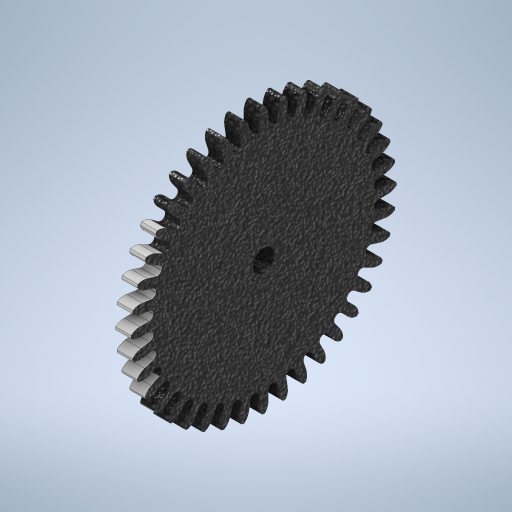
# Autodesk Inventor part: Rear_tubo
Saved by Autodesk Inventor 2024 (Build 280153020, 153B)
## iProperties
Created: 2023-05-22
Part Number: Rear_tubo
Material: Generic
Document SubType Name: Modeling
Designer: Diego
Density: 1 g/cm^3
Appearance: Default
Author: Diego
Autodesk Inventor part; units mm, degrees
ref_plane "YZ Plane" through (0, 0, 0) normal (1, 0, 0) x (0, 1, 0)
ref_plane "XZ Plane" through (0, 0, 0) normal (0, 1, 0) x (-1, 0, 0)
ref_plane "XY Plane" through (0, 0, 0) normal (0, 0, 1) x (1, 0, 0)
sketch "Sketch1" plane through (0, 0, 0) normal (1, 0, 0) x (0, 1, 0)
  circle A0 centre (0, 0) radius 2.5
  arc A1 (-27.9137, 2.1969) -> (-27.9137, -2.1969) centre (0, 0) ccw construction
  line L0 (0, 0) -> (38.0668, 0) construction
  line L1 (0, 0) -> (36.3288, -2.8591) construction
  line L2 (0, 0) -> (35.2598, 2.775) construction
  line L3 (25.9214, 1.02) -> (27.9814, 1.02)
  line L4 (25.9214, -1.02) -> (27.9814, -1.02)
  arc A2 (29.9985, 0.3) -> (27.9814, 1.02) centre (28.0479, -1.9793) ccw
  arc A3 (27.9814, -1.02) -> (29.9985, -0.3) centre (28.0479, 1.9793) ccw
  arc A4 (29.9985, -0.3) -> (29.9985, 0.3) centre (0, 0) ccw
  arc A5 (-29.9985, 0.3) -> (-29.9985, -0.3) centre (0, 0) ccw
  arc A6 (25.9214, -1.02) -> (24.9244, -1.9423) centre (25.9214, -2.02) ccw
  arc A7 (24.9244, 1.9423) -> (25.9214, 1.02) centre (25.9214, 2.02) ccw
  arc A8 (24.3137, 5.8174) -> (25.4427, 5.0624) centre (25.2863, 6.0501) ccw
  line L5 (25.4427, 5.0624) -> (27.4774, 5.3847)
  arc A9 (25.7618, 3.0476) -> (24.9214, 1.9806) centre (25.9183, 2.0599) ccw
  arc A10 (27.7965, 3.3698) -> (29.6761, 4.3965) centre (27.3929, 6.3425) ccw
  arc A11 (29.6761, 4.3965) -> (29.5822, 4.9891) centre (0, 0) ccw
  arc A12 (29.5822, 4.9891) -> (27.4774, 5.3847) centre (28.0122, 2.4328) ccw
  line L6 (25.7618, 3.0476) -> (27.7965, 3.3698)
  arc A13 (23.1043, 9.5493) -> (24.3375, 8.9802) centre (24.0285, 9.9313) ccw
  line L7 (24.3375, 8.9802) -> (26.2967, 9.6168)
  arc A14 (24.9679, 7.0401) -> (24.3048, 5.8548) centre (25.2769, 6.089) ccw
  arc A15 (26.9271, 7.6767) -> (28.623, 8.9847) centre (26.0635, 10.5497) ccw
  arc A16 (28.623, 8.9847) -> (28.4376, 9.5554) centre (0, 0) ccw
  arc A17 (28.4376, 9.5554) -> (26.2967, 9.6168) centre (27.2867, 6.7849) ccw
  line L8 (24.9679, 7.0401) -> (26.9271, 7.6767)
  arc A18 (21.326, 13.0461) -> (22.6331, 12.6769) centre (22.1791, 13.5679) ccw
  line L9 (22.6331, 12.6769) -> (24.4686, 13.6121)
  arc A19 (23.5592, 10.8592) -> (23.0896, 9.5848) centre (24.0132, 9.9682) ccw
  arc A20 (25.3947, 11.7945) -> (26.8651, 13.3517) centre (24.0923, 14.497) ccw
  arc A21 (26.8651, 13.3517) -> (26.5927, 13.8863) centre (0, 0) ccw
  arc A22 (26.5927, 13.8863) -> (24.4686, 13.6121) centre (25.8894, 10.9699) ccw
  line L10 (23.5592, 10.8592) -> (25.3947, 11.7945)
  arc A23 (19.0226, 16.2216) -> (20.3713, 16.0614) centre (19.7835, 16.8704) ccw
  line L11 (20.3713, 16.0614) -> (22.0379, 17.2723)
  arc A24 (21.5704, 14.411) -> (21.306, 13.0789) centre (22.1582, 13.602) ccw
  arc A25 (23.237, 15.6219) -> (24.4456, 17.39) centre (21.5278, 18.0874) ccw
  arc A26 (24.4456, 17.39) -> (24.093, 17.8754) centre (0, 0) ccw
  arc A27 (24.093, 17.8754) -> (22.0379, 17.2723) centre (23.8546, 14.8849) ccw
  line L12 (21.5704, 14.411) -> (23.237, 15.6219)
  arc A28 (16.2508, 18.9977) -> (17.608, 19.0505) centre (16.9009, 19.7576) ccw
  line L13 (17.608, 19.0505) -> (19.0646, 20.5071)
  arc A29 (19.0505, 17.608) -> (18.9977, 16.2508) centre (19.7576, 16.9009) ccw
  arc A30 (20.5071, 19.0646) -> (21.4243, 21) centre (18.4333, 21.2324) ccw
  arc A31 (21.4243, 21) -> (21, 21.4243) centre (0, 0) ccw
  arc A32 (21, 21.4243) -> (19.0646, 20.5071) centre (21.2324, 18.4333) ccw
  line L14 (19.0505, 17.608) -> (20.5071, 19.0646)
  arc A33 (13.0789, 21.306) -> (14.411, 21.5704) centre (13.602, 22.1582) ccw
  line L15 (14.411, 21.5704) -> (15.6219, 23.237)
  arc A34 (16.0614, 20.3713) -> (16.2216, 19.0226) centre (16.8704, 19.7835) ccw
  arc A35 (17.2723, 22.0379) -> (17.8754, 24.093) centre (14.8849, 23.8546) ccw
  arc A36 (17.8754, 24.093) -> (17.39, 24.4456) centre (0, 0) ccw
  arc A37 (17.39, 24.4456) -> (15.6219, 23.237) centre (18.0874, 21.5278) ccw
  line L16 (16.0614, 20.3713) -> (17.2723, 22.0379)
  arc A38 (9.5848, 23.0896) -> (10.8592, 23.5592) centre (9.9682, 24.0132) ccw
  line L17 (10.8592, 23.5592) -> (11.7945, 25.3947)
  arc A39 (12.6769, 22.6331) -> (13.0461, 21.326) centre (13.5679, 22.1791) ccw
  arc A40 (13.6121, 24.4686) -> (13.8863, 26.5927) centre (10.9699, 25.8894) ccw
  arc A41 (13.8863, 26.5927) -> (13.3517, 26.8651) centre (0, 0) ccw
  arc A42 (13.3517, 26.8651) -> (11.7945, 25.3947) centre (14.497, 24.0923) ccw
  line L18 (12.6769, 22.6331) -> (13.6121, 24.4686)
  arc A43 (5.8548, 24.3048) -> (7.0401, 24.9679) centre (6.089, 25.2769) ccw
  line L19 (7.0401, 24.9679) -> (7.6767, 26.9271)
  arc A44 (8.9802, 24.3375) -> (9.5493, 23.1043) centre (9.9313, 24.0285) ccw
  arc A45 (9.6168, 26.2967) -> (9.5554, 28.4376) centre (6.7849, 27.2867) ccw
  arc A46 (9.5554, 28.4376) -> (8.9847, 28.623) centre (0, 0) ccw
  arc A47 (8.9847, 28.623) -> (7.6767, 26.9271) centre (10.5497, 26.0635) ccw
  line L20 (8.9802, 24.3375) -> (9.6168, 26.2967)
  arc A48 (1.9806, 24.9214) -> (3.0476, 25.7618) centre (2.0599, 25.9183) ccw
  line L21 (3.0476, 25.7618) -> (3.3698, 27.7965)
  arc A49 (5.0624, 25.4427) -> (5.8174, 24.3137) centre (6.0501, 25.2863) ccw
  arc A50 (5.3847, 27.4774) -> (4.9891, 29.5822) centre (2.4328, 28.0122) ccw
  arc A51 (4.9891, 29.5822) -> (4.3965, 29.6761) centre (0, 0) ccw
  arc A52 (4.3965, 29.6761) -> (3.3698, 27.7965) centre (6.3425, 27.3929) ccw
  line L22 (5.0624, 25.4427) -> (5.3847, 27.4774)
  arc A53 (-1.9423, 24.9244) -> (-1.02, 25.9214) centre (-2.02, 25.9214) ccw
  line L23 (-1.02, 25.9214) -> (-1.02, 27.9814)
  arc A54 (1.02, 25.9214) -> (1.9423, 24.9244) centre (2.02, 25.9214) ccw
  arc A55 (1.02, 27.9814) -> (0.3, 29.9985) centre (-1.9793, 28.0479) ccw
  arc A56 (0.3, 29.9985) -> (-0.3, 29.9985) centre (0, 0) ccw
  arc A57 (-0.3, 29.9985) -> (-1.02, 27.9814) centre (1.9793, 28.0479) ccw
  line L24 (1.02, 25.9214) -> (1.02, 27.9814)
  arc A58 (-5.8174, 24.3137) -> (-5.0624, 25.4427) centre (-6.0501, 25.2863) ccw
  line L25 (-5.0624, 25.4427) -> (-5.3847, 27.4774)
  arc A59 (-3.0476, 25.7618) -> (-1.9806, 24.9214) centre (-2.0599, 25.9183) ccw
  arc A60 (-3.3698, 27.7965) -> (-4.3965, 29.6761) centre (-6.3425, 27.3929) ccw
  arc A61 (-4.3965, 29.6761) -> (-4.9891, 29.5822) centre (0, 0) ccw
  arc A62 (-4.9891, 29.5822) -> (-5.3847, 27.4774) centre (-2.4328, 28.0122) ccw
  line L26 (-3.0476, 25.7618) -> (-3.3698, 27.7965)
  arc A63 (-9.5493, 23.1043) -> (-8.9802, 24.3375) centre (-9.9313, 24.0285) ccw
  line L27 (-8.9802, 24.3375) -> (-9.6168, 26.2967)
  arc A64 (-7.0401, 24.9679) -> (-5.8548, 24.3048) centre (-6.089, 25.2769) ccw
  arc A65 (-7.6767, 26.9271) -> (-8.9847, 28.623) centre (-10.5497, 26.0635) ccw
  arc A66 (-8.9847, 28.623) -> (-9.5554, 28.4376) centre (0, 0) ccw
  arc A67 (-9.5554, 28.4376) -> (-9.6168, 26.2967) centre (-6.7849, 27.2867) ccw
  line L28 (-7.0401, 24.9679) -> (-7.6767, 26.9271)
  arc A68 (-13.0461, 21.326) -> (-12.6769, 22.6331) centre (-13.5679, 22.1791) ccw
  line L29 (-12.6769, 22.6331) -> (-13.6121, 24.4686)
  arc A69 (-10.8592, 23.5592) -> (-9.5848, 23.0896) centre (-9.9682, 24.0132) ccw
  arc A70 (-11.7945, 25.3947) -> (-13.3517, 26.8651) centre (-14.497, 24.0923) ccw
  arc A71 (-13.3517, 26.8651) -> (-13.8863, 26.5927) centre (0, 0) ccw
  arc A72 (-13.8863, 26.5927) -> (-13.6121, 24.4686) centre (-10.9699, 25.8894) ccw
  line L30 (-10.8592, 23.5592) -> (-11.7945, 25.3947)
  arc A73 (-16.2216, 19.0226) -> (-16.0614, 20.3713) centre (-16.8704, 19.7835) ccw
  line L31 (-16.0614, 20.3713) -> (-17.2723, 22.0379)
  arc A74 (-14.411, 21.5704) -> (-13.0789, 21.306) centre (-13.602, 22.1582) ccw
  arc A75 (-15.6219, 23.237) -> (-17.39, 24.4456) centre (-18.0874, 21.5278) ccw
  arc A76 (-17.39, 24.4456) -> (-17.8754, 24.093) centre (0, 0) ccw
  arc A77 (-17.8754, 24.093) -> (-17.2723, 22.0379) centre (-14.8849, 23.8546) ccw
  line L32 (-14.411, 21.5704) -> (-15.6219, 23.237)
  arc A78 (-18.9977, 16.2508) -> (-19.0505, 17.608) centre (-19.7576, 16.9009) ccw
  line L33 (-19.0505, 17.608) -> (-20.5071, 19.0646)
  arc A79 (-17.608, 19.0505) -> (-16.2508, 18.9977) centre (-16.9009, 19.7576) ccw
  arc A80 (-19.0646, 20.5071) -> (-21, 21.4243) centre (-21.2324, 18.4333) ccw
  arc A81 (-21, 21.4243) -> (-21.4243, 21) centre (0, 0) ccw
  arc A82 (-21.4243, 21) -> (-20.5071, 19.0646) centre (-18.4333, 21.2324) ccw
  line L34 (-17.608, 19.0505) -> (-19.0646, 20.5071)
  arc A83 (-21.306, 13.0789) -> (-21.5704, 14.411) centre (-22.1582, 13.602) ccw
  line L35 (-21.5704, 14.411) -> (-23.237, 15.6219)
  arc A84 (-20.3713, 16.0614) -> (-19.0226, 16.2216) centre (-19.7835, 16.8704) ccw
  arc A85 (-22.0379, 17.2723) -> (-24.093, 17.8754) centre (-23.8546, 14.8849) ccw
  arc A86 (-24.093, 17.8754) -> (-24.4456, 17.39) centre (0, 0) ccw
  arc A87 (-24.4456, 17.39) -> (-23.237, 15.6219) centre (-21.5278, 18.0874) ccw
  line L36 (-20.3713, 16.0614) -> (-22.0379, 17.2723)
  arc A88 (-23.0896, 9.5848) -> (-23.5592, 10.8592) centre (-24.0132, 9.9682) ccw
  line L37 (-23.5592, 10.8592) -> (-25.3947, 11.7945)
  arc A89 (-22.6331, 12.6769) -> (-21.326, 13.0461) centre (-22.1791, 13.5679) ccw
  arc A90 (-24.4686, 13.6121) -> (-26.5927, 13.8863) centre (-25.8894, 10.9699) ccw
  arc A91 (-26.5927, 13.8863) -> (-26.8651, 13.3517) centre (0, 0) ccw
  arc A92 (-26.8651, 13.3517) -> (-25.3947, 11.7945) centre (-24.0923, 14.497) ccw
  line L38 (-22.6331, 12.6769) -> (-24.4686, 13.6121)
  arc A93 (-24.3048, 5.8548) -> (-24.9679, 7.0401) centre (-25.2769, 6.089) ccw
  line L39 (-24.9679, 7.0401) -> (-26.9271, 7.6767)
  arc A94 (-24.3375, 8.9802) -> (-23.1043, 9.5493) centre (-24.0285, 9.9313) ccw
  arc A95 (-26.2967, 9.6168) -> (-28.4376, 9.5554) centre (-27.2867, 6.7849) ccw
  arc A96 (-28.4376, 9.5554) -> (-28.623, 8.9847) centre (0, 0) ccw
  arc A97 (-28.623, 8.9847) -> (-26.9271, 7.6767) centre (-26.0635, 10.5497) ccw
  line L40 (-24.3375, 8.9802) -> (-26.2967, 9.6168)
  arc A98 (-24.9214, 1.9806) -> (-25.7618, 3.0476) centre (-25.9183, 2.0599) ccw
  line L41 (-25.7618, 3.0476) -> (-27.7965, 3.3698)
  arc A99 (-25.4427, 5.0624) -> (-24.3137, 5.8174) centre (-25.2863, 6.0501) ccw
  arc A100 (-27.4774, 5.3847) -> (-29.5822, 4.9891) centre (-28.0122, 2.4328) ccw
  arc A101 (-29.5822, 4.9891) -> (-29.6761, 4.3965) centre (0, 0) ccw
  arc A102 (-29.6761, 4.3965) -> (-27.7965, 3.3698) centre (-27.3929, 6.3425) ccw
  line L42 (-25.4427, 5.0624) -> (-27.4774, 5.3847)
  arc A103 (-24.9244, -1.9423) -> (-25.9214, -1.02) centre (-25.9214, -2.02) ccw
  line L43 (-25.9214, -1.02) -> (-27.9814, -1.02)
  arc A104 (-25.9214, 1.02) -> (-24.9244, 1.9423) centre (-25.9214, 2.02) ccw
  arc A105 (-27.9814, 1.02) -> (-29.9985, 0.3) centre (-28.0479, -1.9793) ccw
  arc A106 (-29.9985, 0.3) -> (-29.9985, -0.3) centre (0, 0) ccw
  arc A107 (-29.9985, -0.3) -> (-27.9814, -1.02) centre (-28.0479, 1.9793) ccw
  line L44 (-25.9214, 1.02) -> (-27.9814, 1.02)
  arc A108 (-24.3137, -5.8174) -> (-25.4427, -5.0624) centre (-25.2863, -6.0501) ccw
  line L45 (-25.4427, -5.0624) -> (-27.4774, -5.3847)
  arc A109 (-25.7618, -3.0476) -> (-24.9214, -1.9806) centre (-25.9183, -2.0599) ccw
  arc A110 (-27.7965, -3.3698) -> (-29.6761, -4.3965) centre (-27.3929, -6.3425) ccw
  arc A111 (-29.6761, -4.3965) -> (-29.5822, -4.9891) centre (0, 0) ccw
  arc A112 (-29.5822, -4.9891) -> (-27.4774, -5.3847) centre (-28.0122, -2.4328) ccw
  line L46 (-25.7618, -3.0476) -> (-27.7965, -3.3698)
  arc A113 (-23.1043, -9.5493) -> (-24.3375, -8.9802) centre (-24.0285, -9.9313) ccw
  line L47 (-24.3375, -8.9802) -> (-26.2967, -9.6168)
  arc A114 (-24.9679, -7.0401) -> (-24.3048, -5.8548) centre (-25.2769, -6.089) ccw
  arc A115 (-26.9271, -7.6767) -> (-28.623, -8.9847) centre (-26.0635, -10.5497) ccw
  arc A116 (-28.623, -8.9847) -> (-28.4376, -9.5554) centre (0, 0) ccw
  arc A117 (-28.4376, -9.5554) -> (-26.2967, -9.6168) centre (-27.2867, -6.7849) ccw
  line L48 (-24.9679, -7.0401) -> (-26.9271, -7.6767)
  arc A118 (-21.326, -13.0461) -> (-22.6331, -12.6769) centre (-22.1791, -13.5679) ccw
  line L49 (-22.6331, -12.6769) -> (-24.4686, -13.6121)
  arc A119 (-23.5592, -10.8592) -> (-23.0896, -9.5848) centre (-24.0132, -9.9682) ccw
  arc A120 (-25.3947, -11.7945) -> (-26.8651, -13.3517) centre (-24.0923, -14.497) ccw
  arc A121 (-26.8651, -13.3517) -> (-26.5927, -13.8863) centre (0, 0) ccw
  arc A122 (-26.5927, -13.8863) -> (-24.4686, -13.6121) centre (-25.8894, -10.9699) ccw
  line L50 (-23.5592, -10.8592) -> (-25.3947, -11.7945)
  arc A123 (-19.0226, -16.2216) -> (-20.3713, -16.0614) centre (-19.7835, -16.8704) ccw
  line L51 (-20.3713, -16.0614) -> (-22.0379, -17.2723)
  arc A124 (-21.5704, -14.411) -> (-21.306, -13.0789) centre (-22.1582, -13.602) ccw
  arc A125 (-23.237, -15.6219) -> (-24.4456, -17.39) centre (-21.5278, -18.0874) ccw
  arc A126 (-24.4456, -17.39) -> (-24.093, -17.8754) centre (0, 0) ccw
  arc A127 (-24.093, -17.8754) -> (-22.0379, -17.2723) centre (-23.8546, -14.8849) ccw
  line L52 (-21.5704, -14.411) -> (-23.237, -15.6219)
  arc A128 (-16.2508, -18.9977) -> (-17.608, -19.0505) centre (-16.9009, -19.7576) ccw
  line L53 (-17.608, -19.0505) -> (-19.0646, -20.5071)
  arc A129 (-19.0505, -17.608) -> (-18.9977, -16.2508) centre (-19.7576, -16.9009) ccw
  arc A130 (-20.5071, -19.0646) -> (-21.4243, -21) centre (-18.4333, -21.2324) ccw
  arc A131 (-21.4243, -21) -> (-21, -21.4243) centre (0, 0) ccw
  arc A132 (-21, -21.4243) -> (-19.0646, -20.5071) centre (-21.2324, -18.4333) ccw
  line L54 (-19.0505, -17.608) -> (-20.5071, -19.0646)
  arc A133 (-13.0789, -21.306) -> (-14.411, -21.5704) centre (-13.602, -22.1582) ccw
  line L55 (-14.411, -21.5704) -> (-15.6219, -23.237)
  arc A134 (-16.0614, -20.3713) -> (-16.2216, -19.0226) centre (-16.8704, -19.7835) ccw
  arc A135 (-17.2723, -22.0379) -> (-17.8754, -24.093) centre (-14.8849, -23.8546) ccw
  arc A136 (-17.8754, -24.093) -> (-17.39, -24.4456) centre (0, 0) ccw
  arc A137 (-17.39, -24.4456) -> (-15.6219, -23.237) centre (-18.0874, -21.5278) ccw
  line L56 (-16.0614, -20.3713) -> (-17.2723, -22.0379)
  arc A138 (-9.5848, -23.0896) -> (-10.8592, -23.5592) centre (-9.9682, -24.0132) ccw
  line L57 (-10.8592, -23.5592) -> (-11.7945, -25.3947)
  arc A139 (-12.6769, -22.6331) -> (-13.0461, -21.326) centre (-13.5679, -22.1791) ccw
  arc A140 (-13.6121, -24.4686) -> (-13.8863, -26.5927) centre (-10.9699, -25.8894) ccw
  arc A141 (-13.8863, -26.5927) -> (-13.3517, -26.8651) centre (0, 0) ccw
  arc A142 (-13.3517, -26.8651) -> (-11.7945, -25.3947) centre (-14.497, -24.0923) ccw
  line L58 (-12.6769, -22.6331) -> (-13.6121, -24.4686)
  arc A143 (-5.8548, -24.3048) -> (-7.0401, -24.9679) centre (-6.089, -25.2769) ccw
  line L59 (-7.0401, -24.9679) -> (-7.6767, -26.9271)
  arc A144 (-8.9802, -24.3375) -> (-9.5493, -23.1043) centre (-9.9313, -24.0285) ccw
  arc A145 (-9.6168, -26.2967) -> (-9.5554, -28.4376) centre (-6.7849, -27.2867) ccw
  arc A146 (-9.5554, -28.4376) -> (-8.9847, -28.623) centre (0, 0) ccw
  arc A147 (-8.9847, -28.623) -> (-7.6767, -26.9271) centre (-10.5497, -26.0635) ccw
  line L60 (-8.9802, -24.3375) -> (-9.6168, -26.2967)
  arc A148 (-1.9806, -24.9214) -> (-3.0476, -25.7618) centre (-2.0599, -25.9183) ccw
  line L61 (-3.0476, -25.7618) -> (-3.3698, -27.7965)
  arc A149 (-5.0624, -25.4427) -> (-5.8174, -24.3137) centre (-6.0501, -25.2863) ccw
  arc A150 (-5.3847, -27.4774) -> (-4.9891, -29.5822) centre (-2.4328, -28.0122) ccw
  arc A151 (-4.9891, -29.5822) -> (-4.3965, -29.6761) centre (0, 0) ccw
  arc A152 (-4.3965, -29.6761) -> (-3.3698, -27.7965) centre (-6.3425, -27.3929) ccw
  line L62 (-5.0624, -25.4427) -> (-5.3847, -27.4774)
  arc A153 (1.9423, -24.9244) -> (1.02, -25.9214) centre (2.02, -25.9214) ccw
  line L63 (1.02, -25.9214) -> (1.02, -27.9814)
  arc A154 (-1.02, -25.9214) -> (-1.9423, -24.9244) centre (-2.02, -25.9214) ccw
  arc A155 (-1.02, -27.9814) -> (-0.3, -29.9985) centre (1.9793, -28.0479) ccw
  arc A156 (-0.3, -29.9985) -> (0.3, -29.9985) centre (0, 0) ccw
  arc A157 (0.3, -29.9985) -> (1.02, -27.9814) centre (-1.9793, -28.0479) ccw
  line L64 (-1.02, -25.9214) -> (-1.02, -27.9814)
  arc A158 (5.8174, -24.3137) -> (5.0624, -25.4427) centre (6.0501, -25.2863) ccw
  line L65 (5.0624, -25.4427) -> (5.3847, -27.4774)
  arc A159 (3.0476, -25.7618) -> (1.9806, -24.9214) centre (2.0599, -25.9183) ccw
  arc A160 (3.3698, -27.7965) -> (4.3965, -29.6761) centre (6.3425, -27.3929) ccw
  arc A161 (4.3965, -29.6761) -> (4.9891, -29.5822) centre (0, 0) ccw
  arc A162 (4.9891, -29.5822) -> (5.3847, -27.4774) centre (2.4328, -28.0122) ccw
  line L66 (3.0476, -25.7618) -> (3.3698, -27.7965)
  arc A163 (9.5493, -23.1043) -> (8.9802, -24.3375) centre (9.9313, -24.0285) ccw
  line L67 (8.9802, -24.3375) -> (9.6168, -26.2967)
  arc A164 (7.0401, -24.9679) -> (5.8548, -24.3048) centre (6.089, -25.2769) ccw
  arc A165 (7.6767, -26.9271) -> (8.9847, -28.623) centre (10.5497, -26.0635) ccw
  arc A166 (8.9847, -28.623) -> (9.5554, -28.4376) centre (0, 0) ccw
  arc A167 (9.5554, -28.4376) -> (9.6168, -26.2967) centre (6.7849, -27.2867) ccw
  line L68 (7.0401, -24.9679) -> (7.6767, -26.9271)
  arc A168 (13.0461, -21.326) -> (12.6769, -22.6331) centre (13.5679, -22.1791) ccw
  line L69 (12.6769, -22.6331) -> (13.6121, -24.4686)
  arc A169 (10.8592, -23.5592) -> (9.5848, -23.0896) centre (9.9682, -24.0132) ccw
  arc A170 (11.7945, -25.3947) -> (13.3517, -26.8651) centre (14.497, -24.0923) ccw
  arc A171 (13.3517, -26.8651) -> (13.8863, -26.5927) centre (0, 0) ccw
  arc A172 (13.8863, -26.5927) -> (13.6121, -24.4686) centre (10.9699, -25.8894) ccw
  line L70 (10.8592, -23.5592) -> (11.7945, -25.3947)
  arc A173 (16.2216, -19.0226) -> (16.0614, -20.3713) centre (16.8704, -19.7835) ccw
  line L71 (16.0614, -20.3713) -> (17.2723, -22.0379)
  arc A174 (14.411, -21.5704) -> (13.0789, -21.306) centre (13.602, -22.1582) ccw
  arc A175 (15.6219, -23.237) -> (17.39, -24.4456) centre (18.0874, -21.5278) ccw
  arc A176 (17.39, -24.4456) -> (17.8754, -24.093) centre (0, 0) ccw
  arc A177 (17.8754, -24.093) -> (17.2723, -22.0379) centre (14.8849, -23.8546) ccw
  line L72 (14.411, -21.5704) -> (15.6219, -23.237)
  arc A178 (18.9977, -16.2508) -> (19.0505, -17.608) centre (19.7576, -16.9009) ccw
  line L73 (19.0505, -17.608) -> (20.5071, -19.0646)
  arc A179 (17.608, -19.0505) -> (16.2508, -18.9977) centre (16.9009, -19.7576) ccw
  arc A180 (19.0646, -20.5071) -> (21, -21.4243) centre (21.2324, -18.4333) ccw
  arc A181 (21, -21.4243) -> (21.4243, -21) centre (0, 0) ccw
  arc A182 (21.4243, -21) -> (20.5071, -19.0646) centre (18.4333, -21.2324) ccw
  line L74 (17.608, -19.0505) -> (19.0646, -20.5071)
  arc A183 (21.306, -13.0789) -> (21.5704, -14.411) centre (22.1582, -13.602) ccw
  line L75 (21.5704, -14.411) -> (23.237, -15.6219)
  arc A184 (20.3713, -16.0614) -> (19.0226, -16.2216) centre (19.7835, -16.8704) ccw
  arc A185 (22.0379, -17.2723) -> (24.093, -17.8754) centre (23.8546, -14.8849) ccw
  arc A186 (24.093, -17.8754) -> (24.4456, -17.39) centre (0, 0) ccw
  arc A187 (24.4456, -17.39) -> (23.237, -15.6219) centre (21.5278, -18.0874) ccw
  line L76 (20.3713, -16.0614) -> (22.0379, -17.2723)
  arc A188 (23.0896, -9.5848) -> (23.5592, -10.8592) centre (24.0132, -9.9682) ccw
  line L77 (23.5592, -10.8592) -> (25.3947, -11.7945)
  arc A189 (22.6331, -12.6769) -> (21.326, -13.0461) centre (22.1791, -13.5679) ccw
  arc A190 (24.4686, -13.6121) -> (26.5927, -13.8863) centre (25.8894, -10.9699) ccw
  arc A191 (26.5927, -13.8863) -> (26.8651, -13.3517) centre (0, 0) ccw
  arc A192 (26.8651, -13.3517) -> (25.3947, -11.7945) centre (24.0923, -14.497) ccw
  line L78 (22.6331, -12.6769) -> (24.4686, -13.6121)
  arc A193 (24.3048, -5.8548) -> (24.9679, -7.0401) centre (25.2769, -6.089) ccw
  line L79 (24.9679, -7.0401) -> (26.9271, -7.6767)
  arc A194 (24.3375, -8.9802) -> (23.1043, -9.5493) centre (24.0285, -9.9313) ccw
  arc A195 (26.2967, -9.6168) -> (28.4376, -9.5554) centre (27.2867, -6.7849) ccw
  arc A196 (28.4376, -9.5554) -> (28.623, -8.9847) centre (0, 0) ccw
  arc A197 (28.623, -8.9847) -> (26.9271, -7.6767) centre (26.0635, -10.5497) ccw
  line L80 (24.3375, -8.9802) -> (26.2967, -9.6168)
  arc A198 (24.9214, -1.9806) -> (25.7618, -3.0476) centre (25.9183, -2.0599) ccw
  line L81 (25.7618, -3.0476) -> (27.7965, -3.3698)
  arc A199 (25.4427, -5.0624) -> (24.3137, -5.8174) centre (25.2863, -6.0501) ccw
  arc A200 (27.4774, -5.3847) -> (29.5822, -4.9891) centre (28.0122, -2.4328) ccw
  arc A201 (29.5822, -4.9891) -> (29.6761, -4.3965) centre (0, 0) ccw
  arc A202 (29.6761, -4.3965) -> (27.7965, -3.3698) centre (27.3929, -6.3425) ccw
  line L82 (25.4427, -5.0624) -> (27.4774, -5.3847)
  arc A203 (24.9244, 1.9423) -> (24.9214, 1.9806) centre (0, 0) ccw
  arc A204 (24.3137, 5.8174) -> (24.3048, 5.8548) centre (0, 0) ccw
  arc A205 (23.1043, 9.5493) -> (23.0896, 9.5848) centre (0, 0) ccw
  arc A206 (21.326, 13.0461) -> (21.306, 13.0789) centre (0, 0) ccw
  arc A207 (19.0226, 16.2216) -> (18.9977, 16.2508) centre (0, 0) ccw
  arc A208 (16.2508, 18.9977) -> (16.2216, 19.0226) centre (0, 0) ccw
  arc A209 (13.0789, 21.306) -> (13.0461, 21.326) centre (0, 0) ccw
  arc A210 (9.5848, 23.0896) -> (9.5493, 23.1043) centre (0, 0) ccw
  arc A211 (5.8548, 24.3048) -> (5.8174, 24.3137) centre (0, 0) ccw
  arc A212 (1.9806, 24.9214) -> (1.9423, 24.9244) centre (0, 0) ccw
  arc A213 (-1.9423, 24.9244) -> (-1.9806, 24.9214) centre (0, 0) ccw
  arc A214 (-5.8174, 24.3137) -> (-5.8548, 24.3048) centre (0, 0) ccw
  arc A215 (-9.5493, 23.1043) -> (-9.5848, 23.0896) centre (0, 0) ccw
  arc A216 (-13.0461, 21.326) -> (-13.0789, 21.306) centre (0, 0) ccw
  arc A217 (-16.2216, 19.0226) -> (-16.2508, 18.9977) centre (0, 0) ccw
  arc A218 (-18.9977, 16.2508) -> (-19.0226, 16.2216) centre (0, 0) ccw
  arc A219 (-21.306, 13.0789) -> (-21.326, 13.0461) centre (0, 0) ccw
  arc A220 (-23.0896, 9.5848) -> (-23.1043, 9.5493) centre (0, 0) ccw
  arc A221 (-24.3048, 5.8548) -> (-24.3137, 5.8174) centre (0, 0) ccw
  arc A222 (-24.9214, 1.9806) -> (-24.9244, 1.9423) centre (0, 0) ccw
  arc A223 (-24.9244, -1.9423) -> (-24.9214, -1.9806) centre (0, 0) ccw
  arc A224 (-24.3137, -5.8174) -> (-24.3048, -5.8548) centre (0, 0) ccw
  arc A225 (-23.1043, -9.5493) -> (-23.0896, -9.5848) centre (0, 0) ccw
  arc A226 (-21.326, -13.0461) -> (-21.306, -13.0789) centre (0, 0) ccw
  arc A227 (-19.0226, -16.2216) -> (-18.9977, -16.2508) centre (0, 0) ccw
  arc A228 (-16.2508, -18.9977) -> (-16.2216, -19.0226) centre (0, 0) ccw
  arc A229 (-13.0789, -21.306) -> (-13.0461, -21.326) centre (0, 0) ccw
  arc A230 (-9.5848, -23.0896) -> (-9.5493, -23.1043) centre (0, 0) ccw
  arc A231 (-5.8548, -24.3048) -> (-5.8174, -24.3137) centre (0, 0) ccw
  arc A232 (-1.9806, -24.9214) -> (-1.9423, -24.9244) centre (0, 0) ccw
  arc A233 (1.9423, -24.9244) -> (1.9806, -24.9214) centre (0, 0) ccw
  arc A234 (24.9214, -1.9806) -> (24.9244, -1.9423) centre (0, 0) ccw
  arc A235 (24.3048, -5.8548) -> (24.3137, -5.8174) centre (0, 0) ccw
  arc A236 (23.0896, -9.5848) -> (23.1043, -9.5493) centre (0, 0) ccw
  arc A237 (21.306, -13.0789) -> (21.326, -13.0461) centre (0, 0) ccw
  arc A238 (18.9977, -16.2508) -> (19.0226, -16.2216) centre (0, 0) ccw
  arc A239 (16.2216, -19.0226) -> (16.2508, -18.9977) centre (0, 0) ccw
  arc A240 (5.8174, -24.3137) -> (5.8548, -24.3048) centre (0, 0) ccw
  arc A241 (9.5493, -23.1043) -> (9.5848, -23.0896) centre (0, 0) ccw
  arc A242 (13.0461, -21.326) -> (13.0789, -21.306) centre (0, 0) ccw
  point P0 (24.9792, 1.02)
  point P1 (24.9792, -1.02)
  point P2 (-27.9814, 1.02)
  dimension "d0" = 5
  dimension "d4" = 9
  dimension "d5" = 4.5
  dimension "d7" = 2.04
  dimension "d8" = 1.02
  dimension "d9" = 0.3
  dimension "d10" = 0.6
  dimension "d11" = 3
  dimension "d12" = 3
  dimension "d13" = 1
  dimension "d16" = 360
  constraints: 404 point on circle, 203 centre point, 166 end point, 4 point on line, 2 coincident, 2 horizontal, 2 tangent, 1 equal radius, 1 parallel, 923 other
  measures "d0" diameter of A0
  measures "d4" angle of L2 L1
  measures "d5" angle of L0 L2
  measures "d7" distance between parallel lines of L4 L3
  measures "d8" distance between parallel lines of L4 L0
  measures "d9" distance from line of L0 A2.start
  measures "d10" distance of A2.start A3.end
  measures "d11" radius of A2
  measures "d12" radius of A3
  measures "d13" radius of A6
extrude "Extrusion2" add sketch "Sketch1" along normal blind 3.5
body "Solid2"
